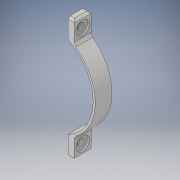
# Autodesk Inventor part: guide_attache
Saved by Autodesk Inventor 2019 (Build 230136000, 136)
## iProperties
Created: 2019-03-20
Part Number: guide_attache
Material: Générique
Document SubType Name: Modeling
Designer: theor
Density: 1 g/cm^3
Appearance: Par défaut
Author: theor
Autodesk Inventor part; units mm, degrees
ref_plane "YZ Plane" through (0, 0, 0) normal (1, 0, 0) x (0, 1, 0)
ref_plane "XZ Plane" through (0, 0, 0) normal (0, 1, 0) x (-1, 0, 0)
ref_plane "XY Plane" through (0, 0, 0) normal (0, 0, 1) x (1, 0, 0)
sketch "Esquisse1" plane through (0, 0, 0) normal (0, 0, 1) x (1, 0, 0)
  arc A0 (22, 0) -> (10, 19.5959) centre (0, 0) ccw
  arc A1 (23, 0) -> (13, 18.9737) centre (0, 0) ccw
  line L0 (13, 18.9737) -> (13, 28.9737)
  line L1 (13, 28.9737) -> (10, 28.9737)
  line L2 (10, 28.9737) -> (10, 19.5959)
  line L3 (23, 0) -> (22, 0)
  dimension "d0" = 1
  dimension "d1" = 22
  dimension "d2" = 10
  dimension "d3" = 3
  dimension "d4" = 10
  constraints: 8 end point, 4 point on circle, 2 centre point, 2 coincident, 2 horizontal, 2 vertical, 1 horizontal alignment
  measures "d0" distance of L3.start L3.end
  measures "d1" radius of A0
  measures "d2" distance of L0.start L0.end
  measures "d3" distance of L0.end L1.end
  measures "d4" distance from line of point (0, 0) L2
extrude "Extrusion1" add sketch "Esquisse1" along normal blind 8
sketch "Esquisse2" plane through (13, 18.9737, 0) normal (1, 0, 0) x (0, 0, -1)
  line L0 (0, 0) -> (0, 10) projected
  line L1 (0, 10) -> (-8, 10) projected
  line L2 (-8, 0) -> (-8, 10) projected
  line L3 (0, 0) -> (-8, 0) projected
  point P0 (0, -18.9737)
  point P1 (-4, 5)
  point P2 (0, 5)
  point P3 (-4, 10)
  constraints: 2 midpoint, 1 horizontal alignment, 1 vertical alignment
hole "Perçage1" at (13, 23.9737, 4) direction (-1, 0, 0) diameter 3.4 depth 3 counterbore diameter 6.5 counterbore depth 1 clearance for "Vis d'assemblage à six pans creux ISO 4762" size "M3" standard "ISO"
chamfer "Chanfrein1" distance 1 angle 45 4 edges at (13, 28.9737, 4) (11.5, 28.9737, 8) (11.5, 28.9737, 0) (13, 18.9737, 4)
mirror "Symétrie1" about plane through (22, 0, 0) normal (0, -1, 0) of "Extrusion1", "Perçage1", "Chanfrein1"
